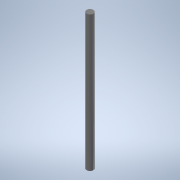
# Autodesk Inventor part: shocks_pin
Saved by Autodesk Inventor 2020 (Build 240168000, 168)
## iProperties
Created: 2015-12-02
Part Number: shocks_pin
Material: Acero inoxidable
Document SubType Name: Modeling
Designer: MIGUEL ANGEL
Density: 8 g/cm^3
Appearance: Semipulido
Author: MIGUEL ANGEL
Autodesk Inventor part; units mm, degrees
ref_plane "YZ Plane" through (0, 0, 0) normal (1, 0, 0) x (0, 1, 0)
ref_plane "XZ Plane" through (0, 0, 0) normal (0, 1, 0) x (-1, 0, 0)
sketch "Boceto1" plane through (0, 0, 0) normal (0, 1, 0) x (-1, 0, 0)
  line L0 (0, 50) -> (0, -50)
  point P0 (0, 0)
  point P1 (0, 0)
  dimension "d0" = 100
  constraints: 2 coincident, 2 end point, 1 midpoint, 1 vertical
  measures "d0" distance of L0.start L0.end
ref_plane "Plano de trabajo1" through (0, 0, 50) normal (0, 0, 1) x (1, 0, 0)
sketch "Boceto2" plane through (0, 0, 50) normal (0, 0, 1) x (1, 0, 0)
  circle A0 centre (0, 0) radius 2.5
  dimension "d2" = 5
  constraints: 1 centre point, 1 coincident
  measures "d2" diameter of A0
sweep "Barrido1" add profiles "Boceto2" path "Boceto1"
